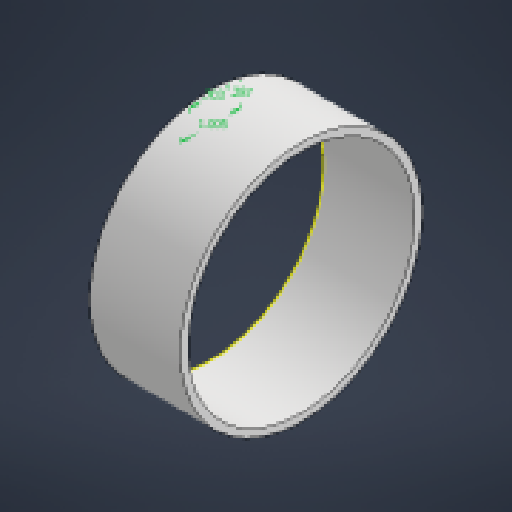
# Autodesk Inventor part: CAST,FLYWHEEL,GRIP
Saved by Autodesk Inventor 2026.1 (Build 301233020, 233B)
## iProperties
Created: 2026-02-02
Part Number: CAST,FLYWHEEL,GRIP
Material: Rubber
Document SubType Name: Modeling
Designer: Owen L
Density: 0.93 g/cm^3
Appearance: Blue - Wall Paint - Glossy
Author: Owen L
Autodesk Inventor part; units mm, degrees
ref_plane "YZ Plane" through (0, 0, 0) normal (1, 0, 0) x (0, 1, 0)
ref_plane "XZ Plane" through (0, 0, 0) normal (0, 1, 0) x (-1, 0, 0)
ref_plane "XY Plane" through (0, 0, 0) normal (0, 0, 1) x (1, 0, 0)
sketch "Sketch1" plane through (0, 0, 0) normal (0, 0, 1) x (1, 0, 0)
  line L0 (-25.4, 50.8) -> (25.4, 50.8)
  line L1 (25.4, 50.8) -> (25.4, 47.625)
  line L2 (25.4, 47.625) -> (-25.4, 47.625)
  line L3 (-25.4, 47.625) -> (-25.4, 50.8)
  line L4 (-35.56, 0) -> (35.56, 0) projected
  point P0 (0, 0)
  point P1 (0, 50.8)
  point P2 (0, 47.625)
  dimension "d0" = 101.6
  dimension "d1" = 3.175
  dimension "d2" = 50.8
  constraints: 8 end point, 2 midpoint, 2 parallel, 2 vertical alignment, 1 horizontal, 1 perpendicular
  measures "d0" diameter of L0 L4
  measures "d1" distance between parallel lines of L0 L2
  measures "d2" distance of L0.start L0.end
revolve "Revolution1" add sketch "Sketch1" angle 360 about axis through (-10, 0, 0) along (1, 0, 0)
sketch "Sketch2" plane through (-25.4, 0, 0) normal (-1, 0, 0) x (0, 0, 1)
  circle A0 centre (0, 0) radius 47.625 projected
  line L0 (-1.016, 47.6142) -> (-2.0955, 45.212)
  line L1 (-2.0955, 45.212) -> (2.0955, 45.212)
  line L2 (2.0955, 45.212) -> (1.016, 47.6142)
  point P0 (0, 45.212)
  dimension "d4" = 4.191
  dimension "d5" = 2.032
  dimension "d6" = 2.413
  constraints: 6 end point, 2 point on circle, 1 equal length, 1 horizontal, 1 midpoint, 1 vertical alignment
  measures "d4" distance of L0.end L1.end
  measures "d5" distance of L2.end L0.start
  measures "d6" distance edge to line of A0 L1
extrude "Extrusion1" add sketch "Sketch2" against normal blind 50.8 contours L2 L1 L0 A0 picked at (0.1129, 46.0159)
pattern_circular "Circular Pattern1" count 40 over 360 about axis through (0, 0, 0) along (1, 0, 0) of "Extrusion1"
body "Solid1"
